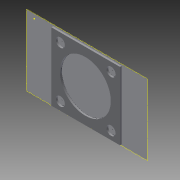
# Autodesk Inventor part: Ball grabber bearing mount2
Saved by Autodesk Inventor 2013 (Build 170138000, 138)
## iProperties
Created: 2014-02-15
Part Number: Ball grabber bearing mount2
Material: Generic
Document SubType Name: Modeling
Designer: robotics
Density: 1 g/cm^3
Author: robotics
Autodesk Inventor part; units mm, degrees
ref_plane "YZ Plane" through (0, 0, 0) normal (1, 0, 0) x (0, 1, 0)
ref_plane "XZ Plane" through (0, 0, 0) normal (0, 1, 0) x (-1, 0, 0)
ref_plane "XY Plane" through (0, 0, 0) normal (0, 0, 1) x (1, 0, 0)
sketch "Sketch1" plane through (0, 0, 0) normal (0, 0, 1) x (1, 0, 0)
  line L0 (-28.9445, 15.5893) -> (396.7701, 15.5893) construction
  line L1 (396.7701, 15.5893) -> (396.7701, -233.6482) construction
  line L2 (396.7701, -233.6482) -> (-28.9445, -233.6482) construction
  line L3 (-28.9445, -233.6482) -> (-28.9445, 15.5893) construction
  line L4 (-26.909, 14.1495) -> (398.8056, 14.1495) construction
  line L5 (398.8056, 14.1495) -> (398.8056, -235.0879) construction
  line L6 (398.8056, -235.0879) -> (-26.909, -235.0879) construction
  line L7 (-26.909, -235.0879) -> (-26.909, 14.1495) construction
  point P0 (0, 0)
  constraints: 4 other
sketch "Sketch2" plane through (0, 0, 0) normal (0, 0, 1) x (1, 0, 0)
  circle A0 centre (97.339, -21.1948) radius 15.8949
  circle A1 centre (275.5323, -21.1948) radius 15.8949
  circle A2 centre (275.5323, -200.173) radius 15.8949
  circle A3 centre (97.339, -200.173) radius 15.8949
  circle A4 centre (185.2582, -110.6839) radius 89.4891
  line L0 (65.9394, 9.4199) -> (306.932, 9.4199)
  line L1 (306.932, 9.4199) -> (306.932, -229.2178)
  line L2 (306.932, -229.2178) -> (65.9394, -229.2178)
  line L3 (65.9394, -229.2178) -> (65.9394, 9.4199)
  point P0 (0, 0)
  constraints: 8 end point, 5 centre point, 2 parallel, 1 horizontal, 1 perpendicular
extrude "Extrusion1" add sketch "Sketch2" along normal blind 6.35
body "Solid1"
